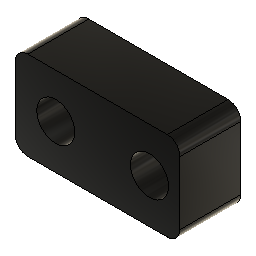
CameraLock v2 (Autodesk Fusion 360 design; units mm, degrees)
Autodesk Fusion 360 part; units mm, degrees
sketch "Sketch1" plane through (0, 0, 0) normal (0, 1, 0) x (1, 0, 0)
  line L0 (-5.5, -3.5) -> (5.5, -3.5)
  line L1 (6.5, -2.5) -> (6.5, 2.5)
  line L2 (5.5, 3.5) -> (-5.5, 3.5)
  line L3 (-6.5, 2.5) -> (-6.5, -2.5)
  line L4 (-6.5, -3.5) -> (6.5, 3.5) construction
  arc A0 (-6.5, -2.5) -> (-5.5, -3.5) centre (-5.5, -2.5) ccw
  arc A1 (5.5, -3.5) -> (6.5, -2.5) centre (5.5, -2.5) ccw
  arc A2 (-5.5, 3.5) -> (-6.5, 2.5) centre (-5.5, 2.5) ccw
  arc A3 (6.5, 2.5) -> (5.5, 3.5) centre (5.5, 2.5) ccw
  line L5 (0, 0) -> (-6.5, 0) construction
  line L6 (0, 0) -> (6.5, 0) construction
  circle A4 centre (4.1, 0) radius 1.5
  circle A5 centre (-3.3, 0) radius 1.5
  line L7 (1.7, -3.5) -> (1.7, 3.5) construction
  point P0 (6.5, -3.5)
  dimension "d1" = 13
  dimension "d2" = 7
  dimension "d3" = 1
  dimension "d4" = 1
  dimension "d5" = 1
  dimension "d6" = 1
  dimension "d7" = 3
  dimension "d8" = 3
  dimension "d11" = 4.8
  dimension "d12" = 2.4
  dimension "d13" = 5
  constraint horizontal L0
  constraint vertical L1
  constraint horizontal L2
  constraint vertical L3
  constraint midpoint L4 L5.start
  constraint coincident L5.start L6.start
  constraint coincident L4.start L3
  constraint coincident L4.start L0
  constraint tangent L3 A0
  constraint tangent L0 A0
  constraint coincident P0 L0
  constraint coincident P0 L1
  constraint tangent L0 A1
  constraint tangent L1 A1
  constraint tangent L3 A2
  constraint tangent L2 A2
  constraint coincident L4.end L2
  constraint coincident L4.end L1
  constraint tangent L2 A3
  constraint tangent L1 A3
  constraint midpoint L3 L5.end
  constraint midpoint L1 L6.end
  constraint coincident L6 A4.centre
  constraint coincident L5 A5.centre
  constraint coincident L0 L7.start
  constraint coincident L2 L7.end
  constraint perpendicular L2 L7
  measures "d1" distance of L4.start P0
  measures "d2" distance of L0 L2
  measures "d3" radius of A0
  measures "d4" radius of A1
  measures "d5" radius of A2
  measures "d6" radius of A3
  measures "d7" diameter of A4
  measures "d8" diameter of A5
  measures "d11" distance of L1 L7
  measures "d12" distance of A4.centre L7
  measures "d13" distance of A5.centre L7
extrude "Extrude1" add sketch "Sketch1" along normal blind 4.8
